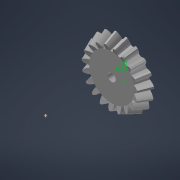
# Autodesk Inventor part: Bevel Gear2
Saved by Autodesk Inventor 2022 (Build 260153000, 153)
## iProperties
CustomPartVersion: 1
Created: 2021-09-12
Part Number: Bevel Gear2
Material: Steel, Mild
Document SubType Name: Modeling
Designer: Andres
Categories: <?xml version="1.0" encoding="UTF-16"?> <MemberInstance><Categories><FamilyTemplate><FamilyTemplateParameter ValueType="xs:double" Id="1" ObjectReferenceKey="da_z" ObjectType="kUserParameterObject"/><FamilyTemplateParameter ValueType="xs:double" Id="2" ObjectReferenceKey="da_b" ObjectType="kUserParameterObject"/><FamilyTemplateParameter ValueType="xs:double" Id="3" ObjectReferenceKey="da_beta" ObjectType="kUserParameterObject"/><FamilyTemplateParameter ValueType="xs:double" Id="4" ObjectReferenceKey="da_dae" ObjectType="kUserParameterObject"/><FamilyTemplateParameter ValueType="xs:double" Id="5" ObjectReferenceKey="da_ve" ObjectType="kUserParameterObject"/><FamilyTemplateParameter ValueType="xs:double" Id="6" ObjectReferenceKey="da_omega" ObjectType="kUserParameterObject"/><FamilyTemplateParameter ValueType="xs:string" Id="7" ObjectReferenceKey="EAIAABAAAAAAHwAAAAAAAIAAAAAAAAAA" ObjectType="83914240" SubObjectId="SurfaceGeometry"/></FamilyTemplate><ParamToTemplateMap><ParamToTemplate CategoryParameter="//CategoryParameter[@InternalName='046C89C9-8512-4d59-83FE-43B91F4F132A']" TemplateParameter="1"/><ParamToTemplate CategoryParameter="//CategoryParameter[@InternalName='2552DF32-E462-4b46-AEBF-C6C7768E72AC']" TemplateParameter="2"/><ParamToTemplate CategoryParameter="//CategoryParameter[@InternalName='C9EE641D-15FC-4fae-A226-E94C4372FDD7']" TemplateParameter="3"/><ParamToTemplate><ParamToTemplate CategoryParameter="//CategoryParameter[@InternalName='00B6519A-459B-49c7-AD84-2E56D39A5744']" ConstantValue="-0.000000"/></ParamToTemplate><ParamToTemplate><ParamToTemplate CategoryParameter="//CategoryParameter[@InternalName='04B31F0E-C7A6-4894-AA32-9629BEFACF47']" ConstantValue="1.000000"/></ParamToTemplate><ParamToTemplate><ParamToTemplate CategoryParameter="//CategoryParameter[@InternalName='43CBEC2E-7847-49e7-A936-2F7889FCB2D9']" ConstantValue="0.200000"/></ParamToTemplate><ParamToTemplate><ParamToTemplate CategoryParameter="//CategoryParameter[@InternalName='B1EFC894-105D-4ebd-86BF-FA20ED196853']" ConstantValue="0.300000"/></ParamToTemplate><ParamToTemplate><ParamToTemplate CategoryParameter="//CategoryParameter[@InternalName='51175063-3D10-4879-93E8-6246FE8B403D']" ConstantValue="2060000000.000000"/></ParamToTemplate><ParamToTemplate><ParamToTemplate CategoryParameter="//CategoryParameter[@InternalName='A3A52E27-4454-46a9-B0BD-C932399B70AF']" ConstantValue="0.300000"/></ParamToTemplate><ParamToTemplate CategoryParameter="//CategoryParameter[@InternalName='2A200944-5A8C-41ca-B96E-8520D2E510F1']" TemplateParameter="4"/><ParamToTemplate><ParamToTemplate CategoryParameter="//CategoryParameter[@InternalName='1A637F62-92C8-44bc-B81F-10802510B579']" ConstantValue="4.406761"/></ParamToTemplate><ParamToTemplate CategoryParameter="//CategoryParameter[@InternalName='B52DD4BE-6863-48fb-BF58-89EF6F9EC65C']" TemplateParameter="5"/><ParamToTemplate><ParamToTemplate CategoryParameter="//CategoryParameter[@InternalName='3956BFF2-84D2-457d-93C2-9B0613DEBA67']" ConstantValue="4.992440"/></ParamToTemplate><ParamToTemplate CategoryParameter="//CategoryParameter[@InternalName='739CFA02-461B-4bf8-8049-181FCAD8B28F']" TemplateParameter="6"/><ParamToTemplate><ParamToTemplate CategoryParameter="//CategoryParameter[@InternalName='A27E999F-E2CE-4481-8A2A-EBF499C4C3C5']" ConstantValue="-0.000000"/></ParamToTemplate><ParamToTemplate><ParamToTemplate CategoryParameter="//CategoryParameter[@InternalName='9E1B4470-B2D3-4ff1-B813-535BB4CDF51A']" ConstantValue="3300000.000000"/></ParamToTemplate><ParamToTemplate><ParamToTemplate CategoryParameter="//CategoryParameter[@InternalName='F8452263-BFF6-458c-9FB1-07C4B99E95CD']" ConstantValue="3700000.000000"/></ParamToTemplate><ParamToTemplate><ParamToTemplate CategoryParameter="//CategoryParameter[@InternalName='3E3BB259-FD49-497f-8171-6EBC954A3479']" ConstantValue="0.000000"/></ParamToTemplate><ParamToTemplate CategoryParameter="//CategoryParameter[@InternalName='27C3BAF2-7550-4e4b-AE2C-0DB134B7D9B7']" TemplateParameter="7"/></ParamToTemplateMap><Category DisplayName="Gear" InternalName="DC85795E-93AB-48d5-8EEE-5A27447B64BD" Mnemonic="Gear"><CategoryParameter DisplayName="z" InternalName="046C89C9-8512-4d59-83FE-43B91F4F132A" Mnemonic="z"/><CategoryParameter DisplayName="b" InternalName="2552DF32-E462-4b46-AEBF-C6C7768E72AC" Mnemonic="b"/><CategoryParameter DisplayName="||b|" InternalName="C9EE641D-15FC-4fae-A226-E94C4372FDD7" Mnemonic="beta"/><CategoryParameter DisplayName="x" InternalName="00B6519A-459B-49c7-AD84-2E56D39A5744" Mnemonic="x"/><CategoryParameter DisplayName="a*" InternalName="04B31F0E-C7A6-4894-AA32-9629BEFACF47" Mnemonic="a"/><CategoryParameter DisplayName="c*" InternalName="43CBEC2E-7847-49e7-A936-2F7889FCB2D9" Mnemonic="c"/><CategoryParameter DisplayName="r|.f|*" InternalName="B1EFC894-105D-4ebd-86BF-FA20ED196853" Mnemonic="rf"/><CategoryParameter DisplayName="E" InternalName="51175063-3D10-4879-93E8-6246FE8B403D" Mnemonic="E"/><CategoryParameter DisplayName="||m|" InternalName="A3A52E27-4454-46a9-B0BD-C932399B70AF" Mnemonic="mi"/><Category DisplayName="BevelGear" InternalName="0C98F69A-0C2B-4791-B2FE-7691BB227E77" Mnemonic="BevelGear"><CategoryParameter DisplayName="d|.ae|" InternalName="2A200944-5A8C-41ca-B96E-8520D2E510F1" Mnemonic="dae"/><CategoryParameter DisplayName="d|.ai|" InternalName="1A637F62-92C8-44bc-B81F-10802510B579" Mnemonic="dai"/><CategoryParameter DisplayName="A|.e|" InternalName="B52DD4BE-6863-48fb-BF58-89EF6F9EC65C" Mnemonic="ve"/><CategoryParameter DisplayName="A|.i|" InternalName="3956BFF2-84D2-457d-93C2-9B0613DEBA67" Mnemonic="vi"/><CategoryParameter DisplayName="||S|" InternalName="739CFA02-461B-4bf8-8049-181FCAD8B28F" Mnemonic="omega"/><CategoryParameter DisplayName="x|.t|" InternalName="A27E999F-E2CE-4481-8A2A-EBF499C4C3C5" Mnemonic="xt"/><CategoryParameter DisplayName="||s||.Flim|" InternalName="9E1B4470-B2D3-4ff1-B813-535BB4CDF51A" Mnemonic="sFlim"/><CategoryParameter DisplayName="||s||.Hlim|" InternalName="F8452263-BFF6-458c-9FB1-07C4B99E95CD" Mnemonic="sHlim"/><CategoryParameter DisplayName="type" InternalName="3E3BB259-FD49-497f-8171-6EBC954A3479" Mnemonic="type"/><CategoryParameter DisplayName="PitchDiameter" InternalName="27C3BAF2-7550-4e4b-AE2C-0DB134B7D9B7" Mnemonic="IDS_PITCHDIAM"/></Category></Category></Categories></MemberInstance>
Mass: 60.9118 g
Surface Area: 34.3074 cm^2
Volume: 7.7496 cm^3
Density: 7.86 g/cm^3
Appearance: Steel
Author: Andres
Autodesk Inventor part; units mm, degrees
ref_plane "XZ Plane" through (0, 0, 0) normal (0, 1, 0) x (-1, 0, 0)
ref_plane "Mesh Plane2" through (0, 0, 0) normal (0.9863613, 0.1645946, 0) x (0, 0, 1)
sketch "Teeth Body Sketch" plane through (0, 0, 0) normal (1, 0, 0) x (0, 1, 0)
  line L0 (0, 0) -> (20.9606, -61.1041) construction
  line L1 (20.9606, -61.1041) -> (26.0745, -59.0799)
  line L2 (26.0745, -59.0799) -> (0, 0) construction
  line L3 (23.75, -60) -> (0, 0) construction
  line L4 (17.7124, -51.635) -> (22.0338, -49.9244)
  line L5 (20.9606, -61.1041) -> (17.7124, -51.635)
  line L6 (26.0745, -59.0799) -> (22.0338, -49.9244)
  line L7 (0, -73.61) -> (0, 12.2683) projected
  line L8 (0, -60) -> (26.0745, -60) construction
  dimension "d0" = 47.5
  dimension "d1" = 41.9212
  dimension "d2" = 52.149
  dimension "d3" = 10
  dimension "d4" = 59.0799
  constraints: 16 end point, 4 point on line, 3 perpendicular, 2 collinear, 1 horizontal alignment, 1 vertical alignment
  measures "d0" diameter of L3.start L7
  measures "d1" diameter of L0.end L7
  measures "d2" diameter of L1.end L7
  measures "d3" distance between parallel lines of L1 L4
  measures "d4" vertical distance of L1.end L0.start
revolve "Teeth Body" add sketch "Teeth Body Sketch" angle 360 about axis through (0, 0, 0) along (0, 0, 1)
ref_plane "Tooth Plane" through (0, 23.75, -60) normal (0, -0.3680485, 0.9298066) x (1, 0, 0)
sketch "Start Sketch" plane through (0, 23.75, -60) normal (0, -0.3680485, 0.9298066) x (1, 0, 0)
  line L0 (0, -41.0848) -> (0, 11.7216) projected
  arc A0 (-1.0841, -3.66) -> (-5.1664, 3.6971) centre (-10.6492, -4.1563) ccw
  arc A1 (5.1664, 3.6971) -> (1.0841, -3.66) centre (10.6492, -4.1563) ccw
  line L1 (-1.0841, -3.66) -> (1.0841, -3.66)
  arc A2 (5.1664, 3.6971) -> (-5.1664, 3.6971) centre (0, -25.5429) ccw
  dimension "d7" = 9.5779
  dimension "d8" = 10.6492
  dimension "d9" = 21.3866
  dimension "d57" = 29.6929
  dimension "d58" = 21.883
  constraints: 6 point on circle, 3 centre point, 3 symmetric about line, 2 end point, 1 coincident, 1 perpendicular, 1 other
  measures "d7" radius of A0
  measures "d8" horizontal distance of point (0, -25.543) A0.centre
  measures "d9" vertical distance of point (0, -25.543) A0.centre
  measures "d57" radius of A2
  measures "d58" distance from line of A2.centre L1
sketch "End Sketch" plane through (0, 19.9683, -50.4462) normal (0, -0.3680485, 0.9298066) x (1, 0, 0)
  line L0 (0, -34.7918) -> (0, 9.9262) projected
  arc A0 (-0.9115, -3.0772) -> (-4.3437, 3.1084) centre (-8.9535, -3.4945) ccw
  arc A1 (4.3437, 3.1084) -> (0.9115, -3.0772) centre (8.9535, -3.4945) ccw
  line L1 (-0.9115, -3.0772) -> (0.9115, -3.0772)
  arc A2 (4.3437, 3.1084) -> (-4.3437, 3.1084) centre (0, -21.4758) ccw
  dimension "d12" = 8.0528
  dimension "d15" = 8.9535
  dimension "d16" = 17.9813
  dimension "d59" = 24.965
  dimension "d60" = 18.3985
  constraints: 6 point on circle, 3 centre point, 3 symmetric about line, 2 end point, 1 coincident, 1 other
  measures "d12" radius of A0
  measures "d15" horizontal distance of A0.centre point (0, -21.476)
  measures "d16" vertical distance of A0.centre point (0, -21.476)
  measures "d59" radius of A2
  measures "d60" distance from line of A2.centre L1
loft "Loft" cut profiles "Start Sketch", "End Sketch"
pattern_circular "Circular Pattern" count 19 over 360 about axis through (0, 0, 0) along (0, 0, 1) of "Loft"
ref_plane "End Plane" through (0, 19.9683, -50.4462) normal (0, -0.3680485, 0.9298066) x (1, 0, 0)
sketch3d "3D Sketch Right"
ref_plane "End Plane Right" through (-2.787, 19.7729, -50.4462) normal (0.0513688, -0.364446, 0.9298066) x (0.9902121, 0.1395707, 0)
sketch "End Sketch Right" plane through (-2.787, 19.7729, -50.4462) normal (0.0513688, -0.364446, 0.9298066) x (0.9902121, 0.1395707, 0)
  arc A0 (-0.9115, -3.0772) -> (-4.3437, 3.1084) centre (-8.9535, -3.4945) ccw
  line L0 (0, -38.8329) -> (0, 13.9672) projected
  arc A1 (4.3437, 3.1084) -> (0.9115, -3.0772) centre (8.9535, -3.4945) ccw
  line L1 (-0.9115, -3.0772) -> (0.9115, -3.0772)
  arc A2 (4.3437, 3.1084) -> (-4.3437, 3.1084) centre (0, -21.4758) ccw
  dimension "d70" = 8.9535
  dimension "d71" = 17.9813
  dimension "d72" = 8.0528
  dimension "d73" = 18.3985
  dimension "d74" = 24.965
  constraints: 6 point on circle, 3 centre point, 3 symmetric about line, 2 end point, 1 coincident, 1 perpendicular, 1 other
  measures "d70" horizontal distance of A2.centre A0.centre
  measures "d71" vertical distance of point (0, -21.476) A0.centre
  measures "d72" radius of A0
  measures "d73" distance from line of point (0, -21.476) L1
  measures "d74" radius of A2
feature "Loft Right" [suppressed]
pattern_circular "Circular Pattern Right" [suppressed]
sketch3d "3D Sketch Left"
ref_plane "End Plane Left" through (2.7838, 19.7729, -50.4453) normal (-0.0513111, -0.3644529, 0.9298071) x (0.9902341, -0.1394144, 0)
sketch "End Sketch Left" plane through (2.7838, 19.7729, -50.4453) normal (-0.0513111, -0.3644529, 0.9298071) x (0.9902341, -0.1394144, 0)
  line L0 (0, -66.897) -> (0, 23.4927) projected
  arc A0 (-0.9115, -3.0771) -> (-4.3437, 3.1085) centre (-8.9535, -3.4944) ccw
  arc A1 (4.3437, 3.1085) -> (0.9115, -3.0771) centre (8.9535, -3.4944) ccw
  line L1 (-0.9115, -3.0771) -> (0.9115, -3.0771)
  ellipse E0 centre (0, -18.3745) end of major axis (22.0338, -18.3745) minor radius 20.4872 projected
  arc A2 (4.3437, 3.1085) -> (-4.3437, 3.1085) centre (0, -21.4757) ccw
  dimension "d56" = 20.4872
  dimension "d30" = 8.0528
  dimension "d31" = 8.9535
  dimension "d32" = 17.9813
  dimension "d61" = 24.965
  dimension "d62" = 18.3985
  constraints: 6 point on circle, 3 centre point, 3 symmetric about line, 2 end point, 1 coincident, 2 other
  measures "d30" radius of A0
  measures "d31" horizontal distance of point (0, -21.476) A0.centre
  measures "d32" vertical distance of A0.centre point (0, -21.476)
  measures "d61" radius of A2
  measures "d62" distance from line of point (0, -21.476) L1
feature "Loft Left" [suppressed]
pattern_circular "Circular Pattern Left" [suppressed]
sketch "Body Sketch" plane through (0, 0, 0) normal (1, 0, 0) x (0, 1, 0)
  line L0 (0, -63.1705) -> (0, -50.3685) projected
  line L1 (20.9606, -61.1041) -> (17.7124, -51.635) projected
  line L2 (17.7124, -51.635) -> (0, -51.635)
  line L3 (20.9606, -61.1041) -> (0, -61.1041)
  constraints: 4 end point, 2 perpendicular, 2 point on line
revolve "Fix Body" add sketch "Body Sketch" angle 360 about axis through (0, 0, 0) along (0, 0, 1)
sketch "Sketch6" plane through (0, 0, 0) normal (1, 0, 0) x (0, 1, 0)
  line L0 (23.75, -60) -> (0, 0) projected
  line L1 (0, -72) -> (0, 12) projected
surface revolve "Pitch Diameter" sketch "Sketch6" angle 360 about axis through (0, 0, 0) along (0, 0, 1) shown no curves L0
sketch "Sketch8" plane through (0, 0, -61.1041) normal (0, 0, -1) x (-1, 0, 0)
  circle A0 centre (0, 0) radius 3.175
  circle A1 centre (0, 0) radius 10
  dimension "d94" = 6.35
  dimension "d95" = 20
  constraints: 2 centre point, 2 coincident
  measures "d94" diameter of A0
  measures "d95" diameter of A1
extrude "Extrusion1" cut sketch "Sketch8" against normal up to surface (9.4692 mm away) contours A0
extrude "Extrusion2" add sketch "Sketch8" along normal blind 8
chamfer "Chamfer1" distance 3 angle 45 1 edges at (10, 0, -61.1041)
equation "\"d0\" = da_de"
equation "\"d1\" = da_dfe"
equation "\"d2\" = da_dae"
equation "\"d3\" = da_b"
equation "\"d4\" = da_ve"
equation "\"d7\" = fd_rr"
equation "\"d8\" = fd_x"
equation "\"d9\" = fd_y"
equation "\"d57\" = 0.5 * fd_dva + 0.3 * da_he"
equation "\"d58\" = 0.5 * fd_dva - 1.12 * da_he"
equation "\"da_teethtype\" = 0"
equation "\"da_b\" = 10"
equation "\"da_de\" = 47.5"
equation "\"da_dae\" = 52.14903"
equation "\"da_dfe\" = 41.92116"
equation "\"da_le\" = 64.52955"
equation "\"da_omega\" = 90deg"
equation "\"da_beta\" = 0"
equation "\"da_delta\" = 21.59531deg"
equation "\"da_alpha\" = 20deg"
equation "\"da_he\" = 5.5"
equation "\"da_ve\" = 59.07988"
equation "\"da_zv\" = 20.434357"
equation "\"fd_loft\" = da_b + 0.05 * da_he"
equation "\"fd_x\" = fd_x1 + fd_x2"
equation "\"fd_y\" = fd_y1 - fd_y2"
equation "\"fd_dd\" = fd_dva - 0.8 * da_he"
equation "\"da_dvw\" = 51.08589"
equation "\"d11\" = fd_loft"
equation "\"da_dm\" = 43.81952"
equation "\"da_x\" = 0"
equation "\"da_m\" = 2.5"
equation "\"d50\" = da_omega"
equation "\"fd_rr\" = 9.577943"
equation "\"fd_dva\" = 56.085892"
equation "\"fd_x1\" = 1.983314"
equation "\"fd_x2\" = 8.665868"
equation "\"fd_y1\" = 25.465831"
equation "\"fd_y2\" = 4.079181"
body "Solid1"
body "Srf1"
